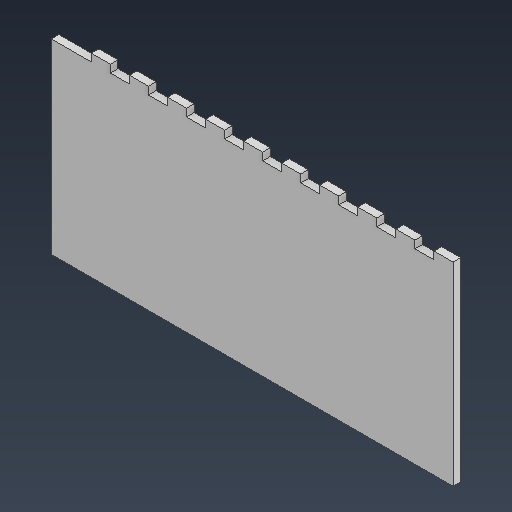
# Autodesk Inventor part: стульчак 2
Saved by Autodesk Inventor 2025 (Build 290162000, 162)
## iProperties
Created: 2025-01-28
Part Number: стульчак 2
Material: Типовые
Document SubType Name: Modeling
Designer: GameHD
Density: 1 g/cm^3
Appearance: По умолчанию
Author: GameHD
Autodesk Inventor part; units mm, degrees
ref_plane "YZ Plane" through (0, 0, 0) normal (1, 0, 0) x (0, 1, 0)
ref_plane "XZ Plane" through (0, 0, 0) normal (0, 1, 0) x (-1, 0, 0)
ref_plane "XY Plane" through (0, 0, 0) normal (0, 0, 1) x (1, 0, 0)
sketch "Эскиз1" plane through (0, 0, 0) normal (0, 0, 1) x (1, 0, 0)
  line L0 (105.5, -51) -> (-105.5, -51)
  line L1 (-105.5, -51) -> (-105.5, 51)
  line L2 (-105.5, 51) -> (105.5, 51)
  line L3 (105.5, 51) -> (105.5, -51)
  line L4 (105.5, -51) -> (-105.5, 51) construction
  line L5 (-105.5, -51) -> (105.5, 51) construction
  line L6 (105.5, 47) -> (-105.5, 47)
  line L7 (105.5, 47) -> (105.5, 51)
  line L8 (105.5, 51) -> (95.5, 51)
  line L9 (95.5, 51) -> (95.5, 47)
  line L10 (95.5, 47) -> (105.5, 47)
  line L11 (85.5, 51) -> (85.5, 47)
  line L12 (95.5, 51) -> (85.5, 51)
  line L13 (95.5, 47) -> (95.5, 51)
  line L14 (85.5, 47) -> (95.5, 47)
  line L15 (75.5, 51) -> (75.5, 47)
  line L16 (85.5, 51) -> (75.5, 51)
  line L17 (85.5, 47) -> (85.5, 51)
  line L18 (75.5, 47) -> (85.5, 47)
  line L19 (65.5, 51) -> (65.5, 47)
  line L20 (75.5, 51) -> (65.5, 51)
  line L21 (75.5, 47) -> (75.5, 51)
  line L22 (65.5, 47) -> (75.5, 47)
  line L23 (55.5, 51) -> (55.5, 47)
  line L24 (65.5, 51) -> (55.5, 51)
  line L25 (65.5, 47) -> (65.5, 51)
  line L26 (55.5, 47) -> (65.5, 47)
  line L27 (45.5, 51) -> (45.5, 47)
  line L28 (55.5, 51) -> (45.5, 51)
  line L29 (55.5, 47) -> (55.5, 51)
  line L30 (45.5, 47) -> (55.5, 47)
  line L31 (35.5, 51) -> (35.5, 47)
  line L32 (45.5, 51) -> (35.5, 51)
  line L33 (45.5, 47) -> (45.5, 51)
  line L34 (35.5, 47) -> (45.5, 47)
  line L35 (25.5, 51) -> (25.5, 47)
  line L36 (35.5, 51) -> (25.5, 51)
  line L37 (35.5, 47) -> (35.5, 51)
  line L38 (25.5, 47) -> (35.5, 47)
  line L39 (15.5, 51) -> (15.5, 47)
  line L40 (25.5, 51) -> (15.5, 51)
  line L41 (25.5, 47) -> (25.5, 51)
  line L42 (15.5, 47) -> (25.5, 47)
  line L43 (5.5, 51) -> (5.5, 47)
  line L44 (15.5, 51) -> (5.5, 51)
  line L45 (15.5, 47) -> (15.5, 51)
  line L46 (5.5, 47) -> (15.5, 47)
  line L47 (-4.5, 51) -> (-4.5, 47)
  line L48 (5.5, 51) -> (-4.5, 51)
  line L49 (5.5, 47) -> (5.5, 51)
  line L50 (-4.5, 47) -> (5.5, 47)
  line L51 (-14.5, 51) -> (-14.5, 47)
  line L52 (-4.5, 51) -> (-14.5, 51)
  line L53 (-4.5, 47) -> (-4.5, 51)
  line L54 (-14.5, 47) -> (-4.5, 47)
  line L55 (-24.5, 51) -> (-24.5, 47)
  line L56 (-14.5, 51) -> (-24.5, 51)
  line L57 (-14.5, 47) -> (-14.5, 51)
  line L58 (-24.5, 47) -> (-14.5, 47)
  line L59 (-34.5, 51) -> (-34.5, 47)
  line L60 (-24.5, 51) -> (-34.5, 51)
  line L61 (-24.5, 47) -> (-24.5, 51)
  line L62 (-34.5, 47) -> (-24.5, 47)
  line L63 (-44.5, 51) -> (-44.5, 47)
  line L64 (-34.5, 51) -> (-44.5, 51)
  line L65 (-34.5, 47) -> (-34.5, 51)
  line L66 (-44.5, 47) -> (-34.5, 47)
  line L67 (-54.5, 51) -> (-54.5, 47)
  line L68 (-44.5, 51) -> (-54.5, 51)
  line L69 (-44.5, 47) -> (-44.5, 51)
  line L70 (-54.5, 47) -> (-44.5, 47)
  line L71 (-64.5, 51) -> (-64.5, 47)
  line L72 (-54.5, 51) -> (-64.5, 51)
  line L73 (-54.5, 47) -> (-54.5, 51)
  line L74 (-64.5, 47) -> (-54.5, 47)
  line L75 (-74.5, 51) -> (-74.5, 47)
  line L76 (-64.5, 51) -> (-74.5, 51)
  line L77 (-64.5, 47) -> (-64.5, 51)
  line L78 (-74.5, 47) -> (-64.5, 47)
  line L79 (-84.5, 51) -> (-84.5, 47)
  line L80 (-74.5, 51) -> (-84.5, 51)
  line L81 (-74.5, 47) -> (-74.5, 51)
  line L82 (-84.5, 47) -> (-74.5, 47)
  line L83 (-84.5, 51) -> (-94.5, 51)
  line L84 (-84.5, 47) -> (-84.5, 51)
  line L85 (-94.5, 47) -> (-84.5, 47)
  line L86 (-94.5, 51) -> (-94.5, 49.2125)
  line L87 (-94.5, 49.2125) -> (-94.5, 47)
  point P0 (0, 0)
  point P1 (-105.5, 47)
  dimension "d0" = 211
  dimension "d1" = 102
  dimension "d2" = 4
  dimension "d3" = 10
  dimension "d4" = 4
  dimension "d5" = 10
  dimension "d6" = 4
  dimension "d7" = 10
  dimension "d8" = 4
  dimension "d9" = 10
  dimension "d10" = 4
  dimension "d11" = 10
  dimension "d12" = 4
  dimension "d13" = 10
  dimension "d14" = 4
  dimension "d15" = 10
  dimension "d16" = 4
  dimension "d17" = 10
  dimension "d18" = 4
  dimension "d19" = 10
  dimension "d20" = 4
  dimension "d21" = 10
  dimension "d22" = 4
  dimension "d23" = 10
  dimension "d24" = 4
  dimension "d25" = 10
  dimension "d26" = 4
  dimension "d27" = 10
  dimension "d28" = 4
  dimension "d29" = 10
  dimension "d30" = 4
  dimension "d31" = 10
  dimension "d32" = 4
  dimension "d33" = 10
  dimension "d34" = 4
  dimension "d35" = 10
  dimension "d36" = 4
  dimension "d37" = 10
  dimension "d38" = 4
  dimension "d39" = 10
  dimension "d40" = 10
  constraints: 174 end point, 40 parallel, 21 perpendicular, 2 horizontal, 2 midpoint, 1 collinear, 3 other
  measures "d0" distance of L1.end L3.start
  measures "d1" distance of L0.end L1.end
  measures "d2" distance of L10.start L8.end
  measures "d3" distance of L8.end L7.end
  measures "d4" distance of L14.start L11.start
  measures "d5" distance of L11.start L12.start
  measures "d6" distance of L15.end L15.start
  measures "d7" distance of L15.start L16.start
  measures "d8" distance of L19.end L19.start
  measures "d9" distance of L19.start L21.end
  measures "d10" distance of L23.end L23.start
  measures "d11" distance of L23.start L24.start
  measures "d12" distance of L27.end L27.start
  measures "d13" distance of L27.start L29.end
  measures "d14" distance of L34.start L32.end
  measures "d15" distance of L32.end L33.end
  measures "d16" distance of L38.start L35.start
  measures "d17" distance of L35.start L36.start
  measures "d18" distance of L39.end L39.start
  measures "d19" distance of L39.start L40.start
  measures "d20" distance of L46.start L44.end
  measures "d21" distance of L44.end L45.end
  measures "d22" distance of L50.start L48.end
  measures "d23" distance of L48.end L48.start
  measures "d24" distance of L54.start L51.start
  measures "d25" distance of L51.start L52.start
  measures "d26" distance of L55.end L55.start
  measures "d27" distance of L55.start L57.end
  measures "d28" distance of L62.start L60.end
  measures "d29" distance of L60.end L61.end
  measures "d30" distance of L66.start L63.start
  measures "d31" distance of L63.start L64.start
  measures "d32" distance of L67.end L67.start
  measures "d33" distance of L67.start L69.end
  measures "d34" distance of L74.start L71.start
  measures "d35" distance of L71.start L72.start
  measures "d36" distance of L78.start L75.start
  measures "d37" distance of L75.start L76.start
  measures "d38" distance of L82.start L79.start
  measures "d39" distance of L79.start L80.start
  measures "d40" distance of L83.end L84.end
extrude "Выдавливание1" add sketch "Эскиз1" along normal blind 4 contours L0 L1 L6 L3 | L6 L9 L2 L3 | L6 L15 L2 L11 | L79 L2 L75 L6 | L6 L23 L2 L19 | L71 L2 L67 L6 | L6 L31 L2 L27 | L63 L2 L59 L6 | L6 L39 L2 L35 | L55 L2 L51 L6 | L6 L47 L2 L43
